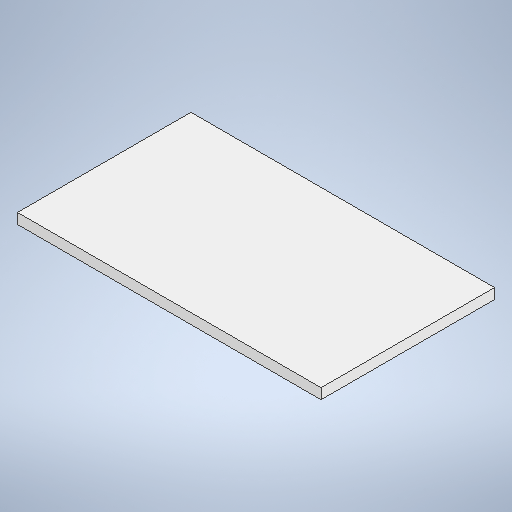
# Autodesk Inventor part: Butcher_Block--1.5_x_24_x_42.75_in
Saved by Autodesk Inventor 2025 (Build 290162000, 162)
## iProperties
Created: 2023-05-06
Part Number: Butcher_Block--1.5_x_24_x_42.75_in
Material: Generic
Document SubType Name: Modeling
Designer: Tom
Density: 1 g/cm^3
Appearance: White
Author: Tom
Autodesk Inventor part; units mm, degrees
ref_plane "YZ Plane" through (0, 0, 0) normal (1, 0, 0) x (0, 1, 0)
ref_plane "XZ Plane" through (0, 0, 0) normal (0, 1, 0) x (-1, 0, 0)
ref_plane "XY Plane" through (0, 0, 0) normal (0, 0, 1) x (1, 0, 0)
sketch "Sketch1" plane through (0, 0, 0) normal (0, 1, 0) x (-1, 0, 0)
  line L0 (0, 0) -> (-1111.25, 0)
  line L1 (-1111.25, 0) -> (-1111.25, -635)
  line L2 (-1111.25, -635) -> (0, -635)
  line L3 (0, -635) -> (0, 0)
  dimension "d6" = 635
  dimension "d7" = 1111.25
  constraints: 8 end point, 2 parallel, 1 coincident, 1 horizontal, 1 perpendicular
  measures "d6" distance of L2.end L0.start
  measures "d7" distance of L1.end L2.end
extrude "Extrusion1" add sketch "Sketch1" along normal blind 38.1
body "Solid1"
